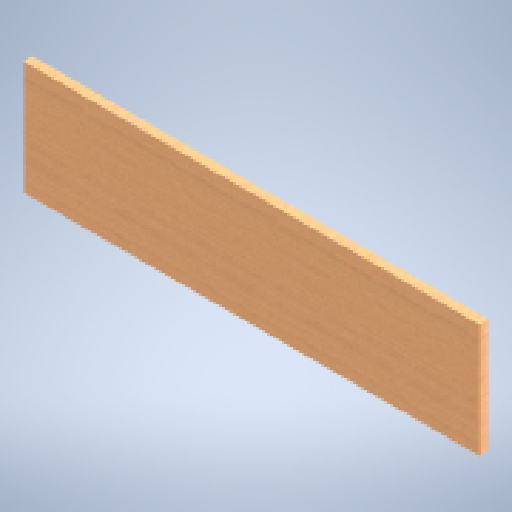
# Autodesk Inventor part: Querseite_Gehäuse
Saved by Autodesk Inventor 2024 (Build 280153000, 153)
## iProperties
Created: 2024-03-12
Part Number: Querseite_Gehäuse
Material: Holz (Kirsche)
Document SubType Name: Modeling
Designer: haniv
Density: 0.63 g/cm^3
Appearance: Kirsche - natur - schwacher Glanz
Author: haniv
Autodesk Inventor part; units mm, degrees
ref_plane "YZ Plane" through (0, 0, 0) normal (1, 0, 0) x (0, 1, 0)
ref_plane "XZ Plane" through (0, 0, 0) normal (0, 1, 0) x (-1, 0, 0)
ref_plane "XY Plane" through (0, 0, 0) normal (0, 0, 1) x (1, 0, 0)
sketch "Skizze1" plane through (0, 0, 0) normal (0, 1, 0) x (-1, 0, 0)
  line L0 (301, 75) -> (-301, 75)
  line L1 (-301, 75) -> (-301, -75)
  line L2 (-301, -75) -> (301, -75)
  line L3 (301, -75) -> (301, 75)
  point P0 (0, 0)
  point P1 (0, -75)
  point P2 (301, 0)
  dimension "d0" = 602
  dimension "d1" = 150
  constraints: 8 end point, 2 midpoint, 2 parallel, 1 horizontal, 1 horizontal alignment, 1 perpendicular, 1 vertical alignment
  measures "d0" distance of L2.end L1.end
  measures "d1" distance of L1.end L0.end
extrude "Extrusion1" add sketch "Skizze1" along normal mid plane 12
sketch "Skizze2" plane through (0, 6, 0) normal (0, 1, 0) x (1, 0, 0)
  line L0 (-301, 75) -> (-301, -75) projected
  line L1 (301, -75) -> (301, 75) projected
  line L2 (-301, -65) -> (301, -65)
  line L3 (301, -65) -> (301, -62.8)
  line L4 (301, -62.8) -> (-301, -62.8)
  line L5 (-301, -62.8) -> (-301, -65)
  line L6 (-301, -75) -> (301, -75) projected
  point P0 (0, 0)
  dimension "d4" = 10
  dimension "d5" = 2.2
  constraints: 8 end point, 2 parallel, 2 point on line, 1 horizontal, 1 perpendicular
  measures "d4" distance between parallel lines of L6 L2
  measures "d5" distance between parallel lines of L4 L2
extrude "Extrusion2" cut sketch "Skizze2" against normal blind 5 contours L4 L1 L2 L0
